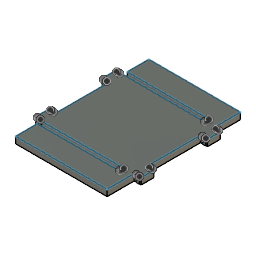
Support - Servo Support with Slots FINAL (Autodesk Fusion 360 design; units mm, degrees)
description: STEP AP242 Edition 2
part number: Servo Support with Slots
Autodesk Fusion 360 part; units mm, degrees
sketch "Sketch1" plane through (0, 0, 3.2) normal (0, 0, 1) x (-1, 0, 0)
  line L0 (-1.6492, -18.6756) -> (36.15, -18.8)
  line L1 (36.15, -18.8) -> (36.15, -18.27)
  line L2 (36.15, -18.27) -> (37.1, -18.27)
  spline S0 degree 3 poles (37.1, -18.27) (37.1, -18.2783) (37.1013, -18.2865) (37.1064, -18.303) (37.1102, -18.3111) (37.1258, -18.3367) (37.1415, -18.3524) (37.1955, -18.3959) (37.2505, -18.4237) (37.4582, -18.4929) (37.6541, -18.52) (38.0459, -18.52) (38.2418, -18.4929) (38.4495, -18.4237) (38.5045, -18.3959) (38.5585, -18.3524) (38.5742, -18.3367) (38.5898, -18.3111) (38.5936, -18.303) (38.5987, -18.2865) (38.6, -18.2783) (38.6, -18.27) knots 0 0 0 0 0.002502 0.002502 0.005177 0.005177 0.01148 0.01148 0.02594 0.02594 0.054889 0.054889 0.083839 0.083839 0.098299 0.098299 0.104601 0.104601 0.107277 0.107277 0.109779 0.109779 0.109779 0.109779
  line L3 (38.6, -18.27) -> (39.35, -18.27)
  line L4 (39.35, -18.27) -> (39.35, -12.37)
  line L5 (39.35, -12.37) -> (38.6, -12.37)
  spline S1 degree 3 poles (38.6, -12.37) (38.6, -12.3617) (38.5987, -12.3535) (38.5936, -12.337) (38.5898, -12.3289) (38.5742, -12.3033) (38.5585, -12.2876) (38.5045, -12.2441) (38.4495, -12.2163) (38.2418, -12.1471) (38.0459, -12.12) (37.6541, -12.12) (37.4582, -12.1471) (37.2505, -12.2163) (37.1955, -12.2441) (37.1415, -12.2876) (37.1258, -12.3033) (37.1102, -12.3289) (37.1064, -12.337) (37.1013, -12.3535) (37.1, -12.3617) (37.1, -12.37) knots 0 0 0 0 0.002502 0.002502 0.005177 0.005177 0.01148 0.01148 0.02594 0.02594 0.054889 0.054889 0.083839 0.083839 0.098299 0.098299 0.104601 0.104601 0.107277 0.107277 0.109779 0.109779 0.109779 0.109779
  line L6 (37.1, -12.37) -> (36.15, -12.37)
  line L7 (36.15, -12.37) -> (36.15, 12.37)
  line L8 (36.15, 12.37) -> (37.1, 12.37)
  spline S2 degree 3 poles (37.1, 12.37) (37.1, 12.3617) (37.1013, 12.3535) (37.1064, 12.337) (37.1102, 12.3289) (37.1258, 12.3033) (37.1415, 12.2876) (37.1955, 12.2441) (37.2505, 12.2163) (37.4582, 12.1471) (37.6541, 12.12) (38.0459, 12.12) (38.2418, 12.1471) (38.4495, 12.2163) (38.5045, 12.2441) (38.5585, 12.2876) (38.5742, 12.3033) (38.5898, 12.3289) (38.5936, 12.337) (38.5987, 12.3535) (38.6, 12.3617) (38.6, 12.37) knots 0 0 0 0 0.002502 0.002502 0.005177 0.005177 0.01148 0.01148 0.02594 0.02594 0.054889 0.054889 0.083839 0.083839 0.098299 0.098299 0.104601 0.104601 0.107277 0.107277 0.109779 0.109779 0.109779 0.109779
  line L9 (38.6, 12.37) -> (39.35, 12.37)
  line L10 (39.35, 12.37) -> (39.35, 18.27)
  line L11 (39.35, 18.27) -> (38.6, 18.27)
  spline S3 degree 3 poles (38.6, 18.27) (38.6, 18.2783) (38.5987, 18.2865) (38.5936, 18.303) (38.5898, 18.3111) (38.5742, 18.3367) (38.5585, 18.3524) (38.5045, 18.3959) (38.4495, 18.4237) (38.2418, 18.4929) (38.0459, 18.52) (37.6541, 18.52) (37.4582, 18.4929) (37.2505, 18.4237) (37.1955, 18.3959) (37.1415, 18.3524) (37.1258, 18.3367) (37.1102, 18.3111) (37.1064, 18.303) (37.1013, 18.2865) (37.1, 18.2783) (37.1, 18.27) knots 0 0 0 0 0.002502 0.002502 0.005177 0.005177 0.01148 0.01148 0.02594 0.02594 0.054889 0.054889 0.083839 0.083839 0.098299 0.098299 0.104601 0.104601 0.107277 0.107277 0.109779 0.109779 0.109779 0.109779
  line L12 (37.1, 18.27) -> (36.15, 18.27)
  line L13 (36.15, 18.27) -> (36.15, 18.8)
  line L14 (36.15, 18.8) -> (-1.6477, 18.5834)
  spline S4 degree 3 poles (-1.6477, 20.5834) (-1.6676, 20.5834) (-1.6874, 20.5809) (-1.7269, 20.5712) (-1.7464, 20.5639) (-1.8065, 20.5344) (-1.8436, 20.5051) (-1.9262, 20.4206) (-1.9832, 20.3423) (-2.1061, 20.0411) (-2.1477, 19.8122) (-2.1477, 19.3546) (-2.1061, 19.1258) (-1.9832, 18.8245) (-1.9262, 18.7462) (-1.8436, 18.6618) (-1.8065, 18.6325) (-1.7464, 18.603) (-1.7269, 18.5957) (-1.6874, 18.5859) (-1.6676, 18.5834) (-1.6477, 18.5834) knots -0.156702 -0.156702 -0.156702 -0.156702 -0.150711 -0.150711 -0.144482 -0.144482 -0.13065 -0.13065 -0.109146 -0.109146 -0.078351 -0.078351 -0.047556 -0.047556 -0.026053 -0.026053 -0.01222 -0.01222 -0.005992 -0.005992 0 0 0 0
  line L15 (-1.6477, 20.5834) -> (36.15, 20.8)
  line L16 (36.15, 20.8) -> (36.15, 30.8)
  line L17 (36.15, 30.8) -> (-6.15, 30.8)
  line L18 (-6.15, 30.8) -> (-6.15, 18.27)
  line L19 (-6.15, 18.27) -> (-7.1, 18.27)
  spline S5 degree 3 poles (-7.1, 18.27) (-7.1, 18.2783) (-7.1013, 18.2865) (-7.1064, 18.303) (-7.1102, 18.3111) (-7.1258, 18.3367) (-7.1415, 18.3524) (-7.1955, 18.3959) (-7.2505, 18.4237) (-7.4582, 18.4929) (-7.6541, 18.52) (-8.0459, 18.52) (-8.2418, 18.4929) (-8.4495, 18.4237) (-8.5045, 18.3959) (-8.5585, 18.3524) (-8.5742, 18.3367) (-8.5898, 18.3111) (-8.5936, 18.303) (-8.5987, 18.2865) (-8.6, 18.2783) (-8.6, 18.27) knots 0 0 0 0 0.002502 0.002502 0.005177 0.005177 0.01148 0.01148 0.02594 0.02594 0.054889 0.054889 0.083839 0.083839 0.098299 0.098299 0.104601 0.104601 0.107277 0.107277 0.109779 0.109779 0.109779 0.109779
  line L20 (-8.6, 18.27) -> (-9.35, 18.27)
  line L21 (-9.35, 18.27) -> (-9.35, 12.37)
  line L22 (-9.35, 12.37) -> (-8.6, 12.37)
  spline S6 degree 3 poles (-8.6, 12.37) (-8.6, 12.3617) (-8.5987, 12.3535) (-8.5936, 12.337) (-8.5898, 12.3289) (-8.5742, 12.3033) (-8.5585, 12.2876) (-8.5045, 12.2441) (-8.4495, 12.2163) (-8.2418, 12.1471) (-8.0459, 12.12) (-7.6541, 12.12) (-7.4582, 12.1471) (-7.2505, 12.2163) (-7.1955, 12.2441) (-7.1415, 12.2876) (-7.1258, 12.3033) (-7.1102, 12.3289) (-7.1064, 12.337) (-7.1013, 12.3535) (-7.1, 12.3617) (-7.1, 12.37) knots 0 0 0 0 0.002502 0.002502 0.005177 0.005177 0.01148 0.01148 0.02594 0.02594 0.054889 0.054889 0.083839 0.083839 0.098299 0.098299 0.104601 0.104601 0.107277 0.107277 0.109779 0.109779 0.109779 0.109779
  line L23 (-7.1, 12.37) -> (-6.15, 12.37)
  line L24 (-6.15, 12.37) -> (-6.15, -12.37)
  line L25 (-6.15, -12.37) -> (-7.1, -12.37)
  spline S7 degree 3 poles (-7.1, -12.37) (-7.1, -12.3617) (-7.1013, -12.3535) (-7.1064, -12.337) (-7.1102, -12.3289) (-7.1258, -12.3033) (-7.1415, -12.2876) (-7.1955, -12.2441) (-7.2505, -12.2163) (-7.4582, -12.1471) (-7.6541, -12.12) (-8.0459, -12.12) (-8.2418, -12.1471) (-8.4495, -12.2163) (-8.5045, -12.2441) (-8.5585, -12.2876) (-8.5742, -12.3033) (-8.5898, -12.3289) (-8.5936, -12.337) (-8.5987, -12.3535) (-8.6, -12.3617) (-8.6, -12.37) knots 0 0 0 0 0.002502 0.002502 0.005177 0.005177 0.01148 0.01148 0.02594 0.02594 0.054889 0.054889 0.083839 0.083839 0.098299 0.098299 0.104601 0.104601 0.107277 0.107277 0.109779 0.109779 0.109779 0.109779
  line L26 (-8.6, -12.37) -> (-9.35, -12.37)
  line L27 (-9.35, -12.37) -> (-9.35, -18.27)
  line L28 (-9.35, -18.27) -> (-8.6, -18.27)
  spline S8 degree 3 poles (-8.6, -18.27) (-8.6, -18.2783) (-8.5987, -18.2865) (-8.5936, -18.303) (-8.5898, -18.3111) (-8.5742, -18.3367) (-8.5585, -18.3524) (-8.5045, -18.3959) (-8.4495, -18.4237) (-8.2418, -18.4929) (-8.0459, -18.52) (-7.6541, -18.52) (-7.4582, -18.4929) (-7.2505, -18.4237) (-7.1955, -18.3959) (-7.1415, -18.3524) (-7.1258, -18.3367) (-7.1102, -18.3111) (-7.1064, -18.303) (-7.1013, -18.2865) (-7.1, -18.2783) (-7.1, -18.27) knots 0 0 0 0 0.002502 0.002502 0.005177 0.005177 0.01148 0.01148 0.02594 0.02594 0.054889 0.054889 0.083839 0.083839 0.098299 0.098299 0.104601 0.104601 0.107277 0.107277 0.109779 0.109779 0.109779 0.109779
  line L29 (-7.1, -18.27) -> (-6.15, -18.27)
  line L30 (-6.15, -18.27) -> (-6.15, -30.8)
  line L31 (-6.15, -30.8) -> (36.15, -30.8)
  line L32 (36.15, -30.8) -> (36.15, -20.8)
  line L33 (36.15, -20.8) -> (-1.6492, -20.6756)
  spline S9 degree 3 poles (-1.6492, -18.6756) (-1.6692, -18.6756) (-1.689, -18.6782) (-1.7285, -18.6879) (-1.748, -18.6952) (-1.808, -18.7247) (-1.8452, -18.754) (-1.9278, -18.8384) (-1.9848, -18.9167) (-2.1077, -19.218) (-2.1492, -19.4468) (-2.1492, -19.9045) (-2.1077, -20.1333) (-1.9848, -20.4345) (-1.9278, -20.5128) (-1.8452, -20.5973) (-1.808, -20.6266) (-1.748, -20.6561) (-1.7285, -20.6634) (-1.689, -20.6731) (-1.6692, -20.6756) (-1.6492, -20.6756) knots -0.156702 -0.156702 -0.156702 -0.156702 -0.150711 -0.150711 -0.144482 -0.144482 -0.13065 -0.13065 -0.109146 -0.109146 -0.078351 -0.078351 -0.047556 -0.047556 -0.026053 -0.026053 -0.01222 -0.01222 -0.005992 -0.005992 0 0 0 0
  line L34 (-7.1, -12.37) -> (-7.1, -12.3617) construction
  line L35 (-7.1, -12.3617) -> (-7.1013, -12.3535) construction
  line L36 (-7.1013, -12.3535) -> (-7.1064, -12.337) construction
  line L37 (-7.1064, -12.337) -> (-7.1102, -12.3289) construction
  line L38 (-7.1102, -12.3289) -> (-7.1258, -12.3033) construction
  line L39 (-7.1258, -12.3033) -> (-7.1415, -12.2876) construction
  line L40 (-7.1415, -12.2876) -> (-7.1955, -12.2441) construction
  line L41 (-7.1955, -12.2441) -> (-7.2505, -12.2163) construction
  line L42 (-7.2505, -12.2163) -> (-7.4582, -12.1471) construction
  line L43 (-7.4582, -12.1471) -> (-7.6541, -12.12) construction
  line L44 (-7.6541, -12.12) -> (-8.0459, -12.12) construction
  line L45 (-8.0459, -12.12) -> (-8.2418, -12.1471) construction
  line L46 (-8.2418, -12.1471) -> (-8.4495, -12.2163) construction
  line L47 (-8.4495, -12.2163) -> (-8.5045, -12.2441) construction
  line L48 (-8.5045, -12.2441) -> (-8.5585, -12.2876) construction
  line L49 (-8.5585, -12.2876) -> (-8.5742, -12.3033) construction
  line L50 (-8.5742, -12.3033) -> (-8.5898, -12.3289) construction
  line L51 (-8.5898, -12.3289) -> (-8.5936, -12.337) construction
  line L52 (-8.5936, -12.337) -> (-8.5987, -12.3535) construction
  line L53 (-8.5987, -12.3535) -> (-8.6, -12.3617) construction
  line L54 (-8.6, -12.3617) -> (-8.6, -12.37) construction
  line L55 (38.6, -12.37) -> (38.6, -12.3617) construction
  line L56 (38.6, -12.3617) -> (38.5987, -12.3535) construction
  line L57 (38.5987, -12.3535) -> (38.5936, -12.337) construction
  line L58 (38.5936, -12.337) -> (38.5898, -12.3289) construction
  line L59 (38.5898, -12.3289) -> (38.5742, -12.3033) construction
  line L60 (38.5742, -12.3033) -> (38.5585, -12.2876) construction
  line L61 (38.5585, -12.2876) -> (38.5045, -12.2441) construction
  line L62 (38.5045, -12.2441) -> (38.4495, -12.2163) construction
  line L63 (38.4495, -12.2163) -> (38.2418, -12.1471) construction
  line L64 (38.2418, -12.1471) -> (38.0459, -12.12) construction
  line L65 (38.0459, -12.12) -> (37.6541, -12.12) construction
  line L66 (37.6541, -12.12) -> (37.4582, -12.1471) construction
  line L67 (37.4582, -12.1471) -> (37.2505, -12.2163) construction
  line L68 (37.2505, -12.2163) -> (37.1955, -12.2441) construction
  line L69 (37.1955, -12.2441) -> (37.1415, -12.2876) construction
  line L70 (37.1415, -12.2876) -> (37.1258, -12.3033) construction
  line L71 (37.1258, -12.3033) -> (37.1102, -12.3289) construction
  line L72 (37.1102, -12.3289) -> (37.1064, -12.337) construction
  line L73 (37.1064, -12.337) -> (37.1013, -12.3535) construction
  line L74 (37.1013, -12.3535) -> (37.1, -12.3617) construction
  line L75 (37.1, -12.3617) -> (37.1, -12.37) construction
  line L76 (-1.6492, -18.6756) -> (-1.6692, -18.6756) construction
  line L77 (-1.6692, -18.6756) -> (-1.689, -18.6782) construction
  line L78 (-1.689, -18.6782) -> (-1.7285, -18.6879) construction
  line L79 (-1.7285, -18.6879) -> (-1.748, -18.6952) construction
  line L80 (-1.748, -18.6952) -> (-1.808, -18.7247) construction
  line L81 (-1.808, -18.7247) -> (-1.8452, -18.754) construction
  line L82 (-1.8452, -18.754) -> (-1.9278, -18.8384) construction
  line L83 (-1.9278, -18.8384) -> (-1.9848, -18.9167) construction
  line L84 (-1.9848, -18.9167) -> (-2.1077, -19.218) construction
  line L85 (-2.1077, -19.218) -> (-2.1492, -19.4468) construction
  line L86 (-2.1492, -19.4468) -> (-2.1492, -19.9045) construction
  line L87 (-2.1492, -19.9045) -> (-2.1077, -20.1333) construction
  line L88 (-2.1077, -20.1333) -> (-1.9848, -20.4345) construction
  line L89 (-1.9848, -20.4345) -> (-1.9278, -20.5128) construction
  line L90 (-1.9278, -20.5128) -> (-1.8452, -20.5973) construction
  line L91 (-1.8452, -20.5973) -> (-1.808, -20.6266) construction
  line L92 (-1.808, -20.6266) -> (-1.748, -20.6561) construction
  line L93 (-1.748, -20.6561) -> (-1.7285, -20.6634) construction
  line L94 (-1.7285, -20.6634) -> (-1.689, -20.6731) construction
  line L95 (-1.689, -20.6731) -> (-1.6692, -20.6756) construction
  line L96 (-1.6692, -20.6756) -> (-1.6492, -20.6756) construction
  line L97 (-8.6, -18.27) -> (-8.6, -18.2783) construction
  line L98 (-8.6, -18.2783) -> (-8.5987, -18.2865) construction
  line L99 (-8.5987, -18.2865) -> (-8.5936, -18.303) construction
  line L100 (-8.5936, -18.303) -> (-8.5898, -18.3111) construction
  line L101 (-8.5898, -18.3111) -> (-8.5742, -18.3367) construction
  line L102 (-8.5742, -18.3367) -> (-8.5585, -18.3524) construction
  line L103 (-8.5585, -18.3524) -> (-8.5045, -18.3959) construction
  line L104 (-8.5045, -18.3959) -> (-8.4495, -18.4237) construction
  line L105 (-8.4495, -18.4237) -> (-8.2418, -18.4929) construction
  line L106 (-8.2418, -18.4929) -> (-8.0459, -18.52) construction
  line L107 (-8.0459, -18.52) -> (-7.6541, -18.52) construction
  line L108 (-7.6541, -18.52) -> (-7.4582, -18.4929) construction
  line L109 (-7.4582, -18.4929) -> (-7.2505, -18.4237) construction
  line L110 (-7.2505, -18.4237) -> (-7.1955, -18.3959) construction
  line L111 (-7.1955, -18.3959) -> (-7.1415, -18.3524) construction
  line L112 (-7.1415, -18.3524) -> (-7.1258, -18.3367) construction
  line L113 (-7.1258, -18.3367) -> (-7.1102, -18.3111) construction
  line L114 (-7.1102, -18.3111) -> (-7.1064, -18.303) construction
  line L115 (-7.1064, -18.303) -> (-7.1013, -18.2865) construction
  line L116 (-7.1013, -18.2865) -> (-7.1, -18.2783) construction
  line L117 (-7.1, -18.2783) -> (-7.1, -18.27) construction
  line L118 (-7.1, 18.27) -> (-7.1, 18.2783) construction
  line L119 (-7.1, 18.2783) -> (-7.1013, 18.2865) construction
  line L120 (-7.1013, 18.2865) -> (-7.1064, 18.303) construction
  line L121 (-7.1064, 18.303) -> (-7.1102, 18.3111) construction
  line L122 (-7.1102, 18.3111) -> (-7.1258, 18.3367) construction
  line L123 (-7.1258, 18.3367) -> (-7.1415, 18.3524) construction
  line L124 (-7.1415, 18.3524) -> (-7.1955, 18.3959) construction
  line L125 (-7.1955, 18.3959) -> (-7.2505, 18.4237) construction
  line L126 (-7.2505, 18.4237) -> (-7.4582, 18.4929) construction
  line L127 (-7.4582, 18.4929) -> (-7.6541, 18.52) construction
  line L128 (-7.6541, 18.52) -> (-8.0459, 18.52) construction
  line L129 (-8.0459, 18.52) -> (-8.2418, 18.4929) construction
  line L130 (-8.2418, 18.4929) -> (-8.4495, 18.4237) construction
  line L131 (-8.4495, 18.4237) -> (-8.5045, 18.3959) construction
  line L132 (-8.5045, 18.3959) -> (-8.5585, 18.3524) construction
  line L133 (-8.5585, 18.3524) -> (-8.5742, 18.3367) construction
  line L134 (-8.5742, 18.3367) -> (-8.5898, 18.3111) construction
  line L135 (-8.5898, 18.3111) -> (-8.5936, 18.303) construction
  line L136 (-8.5936, 18.303) -> (-8.5987, 18.2865) construction
  line L137 (-8.5987, 18.2865) -> (-8.6, 18.2783) construction
  line L138 (-8.6, 18.2783) -> (-8.6, 18.27) construction
  line L139 (37.1, 12.37) -> (37.1, 12.3617) construction
  line L140 (37.1, 12.3617) -> (37.1013, 12.3535) construction
  line L141 (37.1013, 12.3535) -> (37.1064, 12.337) construction
  line L142 (37.1064, 12.337) -> (37.1102, 12.3289) construction
  line L143 (37.1102, 12.3289) -> (37.1258, 12.3033) construction
  line L144 (37.1258, 12.3033) -> (37.1415, 12.2876) construction
  line L145 (37.1415, 12.2876) -> (37.1955, 12.2441) construction
  line L146 (37.1955, 12.2441) -> (37.2505, 12.2163) construction
  line L147 (37.2505, 12.2163) -> (37.4582, 12.1471) construction
  line L148 (37.4582, 12.1471) -> (37.6541, 12.12) construction
  line L149 (37.6541, 12.12) -> (38.0459, 12.12) construction
  line L150 (38.0459, 12.12) -> (38.2418, 12.1471) construction
  line L151 (38.2418, 12.1471) -> (38.4495, 12.2163) construction
  line L152 (38.4495, 12.2163) -> (38.5045, 12.2441) construction
  line L153 (38.5045, 12.2441) -> (38.5585, 12.2876) construction
  line L154 (38.5585, 12.2876) -> (38.5742, 12.3033) construction
  line L155 (38.5742, 12.3033) -> (38.5898, 12.3289) construction
  line L156 (38.5898, 12.3289) -> (38.5936, 12.337) construction
  line L157 (38.5936, 12.337) -> (38.5987, 12.3535) construction
  line L158 (38.5987, 12.3535) -> (38.6, 12.3617) construction
  line L159 (38.6, 12.3617) -> (38.6, 12.37) construction
  line L160 (38.6, 18.27) -> (38.6, 18.2783) construction
  line L161 (38.6, 18.2783) -> (38.5987, 18.2865) construction
  line L162 (38.5987, 18.2865) -> (38.5936, 18.303) construction
  line L163 (38.5936, 18.303) -> (38.5898, 18.3111) construction
  line L164 (38.5898, 18.3111) -> (38.5742, 18.3367) construction
  line L165 (38.5742, 18.3367) -> (38.5585, 18.3524) construction
  line L166 (38.5585, 18.3524) -> (38.5045, 18.3959) construction
  line L167 (38.5045, 18.3959) -> (38.4495, 18.4237) construction
  line L168 (38.4495, 18.4237) -> (38.2418, 18.4929) construction
  line L169 (38.2418, 18.4929) -> (38.0459, 18.52) construction
  line L170 (38.0459, 18.52) -> (37.6541, 18.52) construction
  line L171 (37.6541, 18.52) -> (37.4582, 18.4929) construction
  line L172 (37.4582, 18.4929) -> (37.2505, 18.4237) construction
  line L173 (37.2505, 18.4237) -> (37.1955, 18.3959) construction
  line L174 (37.1955, 18.3959) -> (37.1415, 18.3524) construction
  line L175 (37.1415, 18.3524) -> (37.1258, 18.3367) construction
  line L176 (37.1258, 18.3367) -> (37.1102, 18.3111) construction
  line L177 (37.1102, 18.3111) -> (37.1064, 18.303) construction
  line L178 (37.1064, 18.303) -> (37.1013, 18.2865) construction
  line L179 (37.1013, 18.2865) -> (37.1, 18.2783) construction
  line L180 (37.1, 18.2783) -> (37.1, 18.27) construction
  line L181 (37.1, -18.27) -> (37.1, -18.2783) construction
  line L182 (37.1, -18.2783) -> (37.1013, -18.2865) construction
  line L183 (37.1013, -18.2865) -> (37.1064, -18.303) construction
  line L184 (37.1064, -18.303) -> (37.1102, -18.3111) construction
  line L185 (37.1102, -18.3111) -> (37.1258, -18.3367) construction
  line L186 (37.1258, -18.3367) -> (37.1415, -18.3524) construction
  line L187 (37.1415, -18.3524) -> (37.1955, -18.3959) construction
  line L188 (37.1955, -18.3959) -> (37.2505, -18.4237) construction
  line L189 (37.2505, -18.4237) -> (37.4582, -18.4929) construction
  line L190 (37.4582, -18.4929) -> (37.6541, -18.52) construction
  line L191 (37.6541, -18.52) -> (38.0459, -18.52) construction
  line L192 (38.0459, -18.52) -> (38.2418, -18.4929) construction
  line L193 (38.2418, -18.4929) -> (38.4495, -18.4237) construction
  line L194 (38.4495, -18.4237) -> (38.5045, -18.3959) construction
  line L195 (38.5045, -18.3959) -> (38.5585, -18.3524) construction
  line L196 (38.5585, -18.3524) -> (38.5742, -18.3367) construction
  line L197 (38.5742, -18.3367) -> (38.5898, -18.3111) construction
  line L198 (38.5898, -18.3111) -> (38.5936, -18.303) construction
  line L199 (38.5936, -18.303) -> (38.5987, -18.2865) construction
  line L200 (38.5987, -18.2865) -> (38.6, -18.2783) construction
  line L201 (38.6, -18.2783) -> (38.6, -18.27) construction
  line L202 (-1.6477, 20.5834) -> (-1.6676, 20.5834) construction
  line L203 (-1.6676, 20.5834) -> (-1.6874, 20.5809) construction
  line L204 (-1.6874, 20.5809) -> (-1.7269, 20.5712) construction
  line L205 (-1.7269, 20.5712) -> (-1.7464, 20.5639) construction
  line L206 (-1.7464, 20.5639) -> (-1.8065, 20.5344) construction
  line L207 (-1.8065, 20.5344) -> (-1.8436, 20.5051) construction
  line L208 (-1.8436, 20.5051) -> (-1.9262, 20.4206) construction
  line L209 (-1.9262, 20.4206) -> (-1.9832, 20.3423) construction
  line L210 (-1.9832, 20.3423) -> (-2.1061, 20.0411) construction
  line L211 (-2.1061, 20.0411) -> (-2.1477, 19.8122) construction
  line L212 (-2.1477, 19.8122) -> (-2.1477, 19.3546) construction
  line L213 (-2.1477, 19.3546) -> (-2.1061, 19.1258) construction
  line L214 (-2.1061, 19.1258) -> (-1.9832, 18.8245) construction
  line L215 (-1.9832, 18.8245) -> (-1.9262, 18.7462) construction
  line L216 (-1.9262, 18.7462) -> (-1.8436, 18.6618) construction
  line L217 (-1.8436, 18.6618) -> (-1.8065, 18.6325) construction
  line L218 (-1.8065, 18.6325) -> (-1.7464, 18.603) construction
  line L219 (-1.7464, 18.603) -> (-1.7269, 18.5957) construction
  line L220 (-1.7269, 18.5957) -> (-1.6874, 18.5859) construction
  line L221 (-1.6874, 18.5859) -> (-1.6676, 18.5834) construction
  line L222 (-1.6676, 18.5834) -> (-1.6477, 18.5834) construction
  line L223 (-8.6, 12.37) -> (-8.6, 12.3617) construction
  line L224 (-8.6, 12.3617) -> (-8.5987, 12.3535) construction
  line L225 (-8.5987, 12.3535) -> (-8.5936, 12.337) construction
  line L226 (-8.5936, 12.337) -> (-8.5898, 12.3289) construction
  line L227 (-8.5898, 12.3289) -> (-8.5742, 12.3033) construction
  line L228 (-8.5742, 12.3033) -> (-8.5585, 12.2876) construction
  line L229 (-8.5585, 12.2876) -> (-8.5045, 12.2441) construction
  line L230 (-8.5045, 12.2441) -> (-8.4495, 12.2163) construction
  line L231 (-8.4495, 12.2163) -> (-8.2418, 12.1471) construction
  line L232 (-8.2418, 12.1471) -> (-8.0459, 12.12) construction
  line L233 (-8.0459, 12.12) -> (-7.6541, 12.12) construction
  line L234 (-7.6541, 12.12) -> (-7.4582, 12.1471) construction
  line L235 (-7.4582, 12.1471) -> (-7.2505, 12.2163) construction
  line L236 (-7.2505, 12.2163) -> (-7.1955, 12.2441) construction
  line L237 (-7.1955, 12.2441) -> (-7.1415, 12.2876) construction
  line L238 (-7.1415, 12.2876) -> (-7.1258, 12.3033) construction
  line L239 (-7.1258, 12.3033) -> (-7.1102, 12.3289) construction
  line L240 (-7.1102, 12.3289) -> (-7.1064, 12.337) construction
  line L241 (-7.1064, 12.337) -> (-7.1013, 12.3535) construction
  line L242 (-7.1013, 12.3535) -> (-7.1, 12.3617) construction
  line L243 (-7.1, 12.3617) -> (-7.1, 12.37) construction
extrude "Extrude1" add sketch "Sketch1" against normal blind 3
